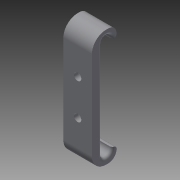
# Autodesk Inventor part: HolderMid
Saved by Autodesk Inventor 2015 (Build 190159000, 159)
## iProperties
Created: 2017-03-07
Part Number: HolderMid
Material: Generic
Document SubType Name: Modeling
Designer: 1esh9
Density: 1 g/cm^3
Appearance: Default
Author: 1esh9
Autodesk Inventor part; units mm, degrees
ref_plane "YZ Plane" through (0, 0, 0) normal (1, 0, 0) x (0, 1, 0)
ref_plane "XZ Plane" through (0, 0, 0) normal (0, 1, 0) x (-1, 0, 0)
ref_plane "XY Plane" through (0, 0, 0) normal (0, 0, 1) x (1, 0, 0)
sketch "Sketch1" plane through (0, 0, 0) normal (0, 1, 0) x (-1, 0, 0)
  circle A0 centre (0, 12.5) radius 2.6
  circle A1 centre (0, -12.5) radius 2.6
  circle A2 centre (0, 12.5) radius 4.75
  circle A3 centre (0, -12.5) radius 4.75
  circle A4 centre (0, 12.5) radius 7.5
  circle A5 centre (0, -12.5) radius 7.5
  line L0 (7.5, 12.5) -> (7.5, -12.5)
  line L1 (-7.5, -12.5) -> (-7.5, 12.5)
  line L2 (0, 12.5) -> (0, -12.5) construction
  line L3 (7.5, -12.5) -> (7.5, 12.5)
  line L4 (-10, 41) -> (10, 41)
  line L5 (10, 41) -> (10, -41)
  line L6 (10, -41) -> (-10, -41)
  line L7 (-10, -41) -> (-10, 41)
  point P0 (0, 0)
  dimension "d0" = 5.2
  dimension "d1" = 5.2
  dimension "d2" = 25
  dimension "d3" = 12.5
  dimension "d6" = 9.5
  dimension "d7" = 9.5
  dimension "d8" = 15
  dimension "d9" = 15
  dimension "d19" = 20
  dimension "d20" = 82
  dimension "d21" = 41
  dimension "d38" = 10
  constraints: 16 end point, 6 centre point, 4 coincident, 4 point on circle, 4 tangent, 2 parallel, 1 horizontal, 1 midpoint, 1 perpendicular, 1 vertical
  measures "d0" diameter of A0
  measures "d1" diameter of A1
  measures "d2" distance of A1.centre A0.centre
  measures "d3" distance of point (0, 0) A1.centre
  measures "d6" diameter of A2
  measures "d7" diameter of A3
  measures "d8" diameter of A4
  measures "d9" diameter of A5
  measures "d19" distance of L5.end L6.end
  measures "d20" distance of L5.end L4.end
  measures "d21" distance from line of point (0, 0) L4
  measures "d38" distance from line of point (0, 0) L7
extrude "Extrusion1" add sketch "Sketch1" along normal blind 3 contours A2 | A3
extrude "Extrusion2" add sketch "Sketch1" along normal blind 7 contours A4 | L0 A5 L1 A4 | A5 | L4 L5 L6 L7
sketch "Sketch2" plane through (0, 7, 0) normal (0, 1, 0) x (1, 0, 0)
  circle A0 centre (0, 12.5) radius 4.75 projected
  circle A1 centre (0, -12.5) radius 4.75 projected
  line L0 (-10, -41) -> (10, -41) projected
  line L1 (10, -41) -> (10, 41) projected
  line L2 (10, 41) -> (-10, 41) projected
  line L3 (-10, 41) -> (-10, -41) projected
  line L4 (10, 41) -> (10, -41) projected
  line L5 (10, -37) -> (-10, -37)
  line L6 (10, 37) -> (-10, 37)
  point P0 (0, 0)
  dimension "d24" = 4
  dimension "d25" = 4
  constraints: 4 end point, 4 point on line, 2 perpendicular
  measures "d24" distance between parallel lines of L0 L5
  measures "d25" distance between parallel lines of L2 L6
extrude "Extrusion3" add sketch "Sketch2" along normal blind 7.4 contours L3 L5 L1 L0 | L3 L2 L1 L6
sketch "Sketch3" plane through (0, 14.4, 0) normal (0, 1, 0) x (1, 0, 0)
  line L0 (10, 41) -> (-10, 41) projected
  line L1 (-10, 41) -> (-10, 37) projected
  line L2 (-10, -41) -> (10, -41) projected
  line L3 (10, 37) -> (10, 41) projected
  line L4 (-10, 37) -> (10, 37) projected
  line L5 (10, -41) -> (10, -37) projected
  line L6 (10, -37) -> (-10, -37) projected
  line L7 (-10, -37) -> (-10, -41) projected
  line L8 (-10, -41) -> (10, -41)
  line L9 (10, -41) -> (10, -33)
  line L10 (10, -33) -> (-10, -33)
  line L11 (-10, -33) -> (-10, -41)
  line L12 (10, -37) -> (10, 37) projected
  line L13 (-10, 41) -> (10, 41)
  line L14 (10, 41) -> (10, 33)
  line L15 (10, 33) -> (-10, 33)
  line L16 (-10, 33) -> (-10, 41)
  dimension "d39" = 4
  dimension "d40" = 4
  constraints: 16 end point, 4 parallel, 2 horizontal, 2 perpendicular, 1 point on line
  measures "d39" distance between parallel lines of L6 L10
  measures "d40" distance between parallel lines of L4 L15
extrude "Extrusion4" add sketch "Sketch3" along normal blind 3
fillet "Fillet4" radius 3 2 edges at (0, 7, 37) (0, 7, -37)
fillet "Fillet5" radius 4 2 edges at (0, 14.4, -37) (0, 14.4, 37)
fillet "Fillet6" radius 2 2 edges at (0, 17.4, 33) (0, 17.4, -33)
fillet "Fillet7" radius 10 2 edges at (0, 0, 41) (0, 0, -41)
fillet "Fillet8" radius 6 2 edges at (0, 17.4, 41) (0, 17.4, -41)
fillet "Fillet9" radius 2 18 edges at (10, 7.8787, -36.1213) (10, 10.2001, -37) (10, 14.4, -33.0001) (10, 13.2285, -35.8285) (10, 7.8787, 36.1213) (10, 10.2001, 37) (10, 14.4, 33.0001) (10, 13.2285, 35.8285) (10, 7, 0) (-10, 7.8787, 36.1213) (-10, 10.2001, 37) (-10, 14.4, 33.0001) (-10, 13.2285, 35.8285) (-10, 7.8787, -36.1213) (-10, 10.2001, -37) (-10, 14.4, -33.0001) (-10, 13.2285, -35.8285) (-10, 7, 0)
equation "\"d3\" = 0.5 * d2"
equation "\"d21\" = 0.5 * d20"
equation "\"d38\" = 0.5 * d19"
body "Solid1"
